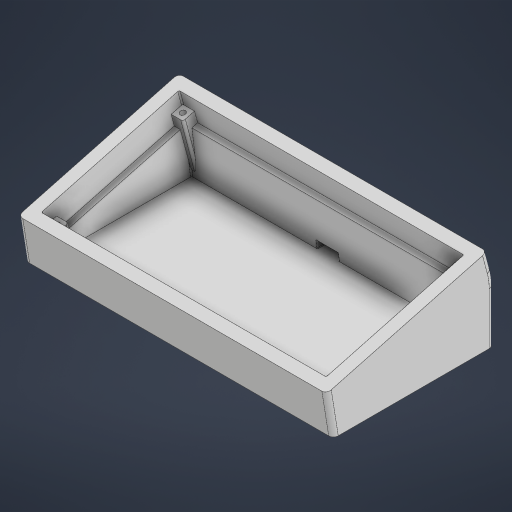
# Autodesk Inventor part: case
Saved by Autodesk Inventor 2024.2 (Build 282272000, 272)
## iProperties
Created: 2024-08-19
Part Number: case
Material: Generic
Document SubType Name: Modeling
Designer: Moe
Density: 1 g/cm^3
Appearance: Default
Author: Moe
Autodesk Inventor part; units mm, degrees
ref_plane "YZ Plane" through (0, 0, 0) normal (1, 0, 0) x (0, 1, 0)
ref_plane "XZ Plane" through (0, 0, 0) normal (0, 1, 0) x (-1, 0, 0)
sketch "Sketch1" plane through (0, 0, 0) normal (1, 0, 0) x (0, 1, 0)
  line L0 (0, 0) -> (7, 0)
  line L1 (7, 0) -> (25.1173, -67.6148)
  line L2 (25.1173, -67.6148) -> (0, -67.6148)
  line L3 (0, -67.6148) -> (0, 0)
  dimension "d0" = 7
  dimension "d1" = 70
  dimension "d2" = 105
  constraints: 8 end point, 1 horizontal, 1 parallel, 1 perpendicular
  measures "d0" distance of L0.start L0.end
  measures "d1" distance of L0.end L1.end
  measures "d2" angle of L0 L1
extrude "Extrusion1" add sketch "Sketch1" along normal blind 130
ref_plane "Work Plane1" through (0, 25, -67.6148) normal (0, -1, 0) x (1, 0, 0)
sketch "Sketch3" plane through (0, 7, 0) normal (0, 0.9659258, 0.258819) x (1, 0, 0)
  line L0 (5, 65) -> (125, 65)
  line L1 (125, 65) -> (125, 5)
  line L2 (125, 5) -> (5, 5)
  line L3 (5, 5) -> (5, 65)
  line L4 (0, 70) -> (130, 70) projected
  line L5 (0, 0) -> (130, 0) projected
  line L6 (0, 70) -> (0, 0) projected
  line L7 (130, 70) -> (130, 0) projected
  line L8 (5, 5) -> (10, 5)
  line L9 (10, 5) -> (10, 10)
  line L10 (10, 10) -> (5, 10)
  line L11 (5, 10) -> (5, 5)
  line L12 (5, 65) -> (10, 65)
  line L13 (10, 65) -> (10, 60)
  line L14 (10, 60) -> (5, 60)
  line L15 (5, 60) -> (5, 65)
  line L16 (125, 65) -> (120, 65)
  line L17 (120, 65) -> (120, 60)
  line L18 (120, 60) -> (125, 60)
  line L19 (125, 60) -> (125, 65)
  line L20 (125, 5) -> (120, 5)
  line L21 (120, 5) -> (120, 10)
  line L22 (120, 10) -> (125, 10)
  line L23 (125, 10) -> (125, 5)
  point P0 (0, -1.8117)
  point P1 (10, 5)
  dimension "d6" = 5
  dimension "d7" = 5
  dimension "d8" = 5
  dimension "d9" = 5
  dimension "d10" = 5
  dimension "d11" = 5
  dimension "d12" = 5
  dimension "d13" = 5
  dimension "d14" = 5
  dimension "d15" = 5
  dimension "d16" = 5
  dimension "d17" = 5
  constraints: 40 end point, 10 parallel, 5 horizontal, 5 perpendicular
  measures "d6" distance between parallel lines of L4 L0
  measures "d7" distance between parallel lines of L2 L5
  measures "d8" distance between parallel lines of L6 L3
  measures "d9" distance between parallel lines of L7 L1
  measures "d10" distance of L10.end L9.end
  measures "d11" distance of L9.end L8.end
  measures "d12" distance of L13.end L14.end
  measures "d13" distance of L12.end L13.end
  measures "d14" distance of L18.end L17.end
  measures "d15" distance of L17.end L16.end
  measures "d16" distance of L21.end L22.end
  measures "d17" distance of L20.end L21.end
sketch "Sketch4" plane through (0, 25, -67.6148) normal (0, -1, 0) x (1, 0, 0)
  line L0 (5, 57.9555) -> (5, 62.7852) projected
  line L1 (5, 62.7852) -> (5, 4.8296) projected
  line L2 (5, 62.7852) -> (10, 62.7852) projected
  line L3 (125, 62.7852) -> (5, 62.7852) projected
  line L4 (5, 4.8296) -> (125, 4.8296) projected
  line L5 (125, 4.8296) -> (125, 62.7852) projected
  point P0 (0, 67.6148)
extrude "Extrusion3" cut sketch "Sketch4" along normal blind 22
extrude "Extrusion4" add sketch "Sketch3" against normal blind 8 contours L10 L9 L2 L3 | L1 L2 L21 L22
sketch "Sketch5" plane through (10, 3, -6.2482) normal (1, 0, 0) x (0, 0, -1)
  line L0 (5.1764, 0) -> (0, 0) projected
  line L1 (0, 0) -> (-1.4185, 0)
  line L2 (-1.4185, 5.2941) -> (0, 0) projected
  line L3 (-1.4185, 0) -> (-1.4185, 5.2941)
  line L4 (-1.4185, 5.2941) -> (0, 0)
  point P0 (-6.2482, -3)
  constraints: 6 end point, 1 perpendicular
extrude "Extrusion5" add sketch "Sketch5" against normal blind 8
extrude "Extrusion6" add sketch "Sketch5" along normal blind 110
extrude "Extrusion7" add sketch "Sketch3" against normal blind 18 contours L0 L13 L14 L3 | L0 L1 L18 L17
extrude "Extrusion8" add sketch "Sketch3" along normal blind 5.1 contours L0 L13 L14 L3 | L0 L1 L18 L17 | L10 L9 L2 L3 | L1 L2 L21 L22
sketch "Sketch6" plane through (0, 7, 0) normal (0, 0.9659258, 0.258819) x (1, 0, 0)
  line L0 (7.5, 62.5) -> (122.5, 62.5)
  line L1 (122.5, 62.5) -> (122.5, 7.5)
  line L2 (122.5, 7.5) -> (7.5, 7.5)
  line L3 (7.5, 7.5) -> (7.5, 62.5)
  line L4 (10, 65) -> (120, 65) projected
  line L5 (5, 10) -> (5, 60) projected
  line L6 (120, 5) -> (10, 5) projected
  line L7 (125, 60) -> (125, 10) projected
  line L8 (5, 65) -> (5, 60) projected
  line L9 (120, 5) -> (125, 5) projected
  line L10 (5, 65) -> (125, 65)
  line L11 (125, 65) -> (125, 5)
  line L12 (125, 5) -> (5, 5)
  line L13 (5, 5) -> (5, 65)
  point P0 (0, -1.8117)
  point P1 (10, 5)
  point P2 (125, 10)
  dimension "d32" = 2.5
  dimension "d33" = 2.5
  dimension "d34" = 2.5
  dimension "d35" = 2.5
  constraints: 16 end point, 4 parallel, 2 horizontal, 2 perpendicular
  measures "d32" distance between parallel lines of L4 L0
  measures "d33" distance between parallel lines of L5 L3
  measures "d34" distance between parallel lines of L6 L2
  measures "d35" distance between parallel lines of L7 L1
extrude "Extrusion9" add sketch "Sketch6" against normal blind 8
sketch "Sketch7" plane through (5, 3, -62.7852) normal (1, 0, 0) x (0, 0, -1)
  line L0 (-2.7591, 11.8017) -> (-46.8038, 0) projected
  line L1 (-46.8038, 0) -> (0, 0) projected
  line L2 (0, 2.1883) -> (0, 0) projected
  line L3 (0, 2.1883) -> (-0.1709, 2.1425) projected
  line L4 (-0.1709, 2.1425) -> (-2.7591, 11.8017) projected
  point P0 (-62.7852, -3)
extrude "Extrusion10" add sketch "Sketch7" along normal blind 2.5
sketch "Sketch8" plane through (10, 5.1883, -62.7852) normal (1, 0, 0) x (0, 0, -1)
  line L0 (-0.3443, 10.2605) -> (-2.4148, 17.9879) projected
  line L1 (-2.4148, 17.9879) -> (0, -2.1883)
  line L2 (0, 10.3528) -> (-0.3443, 10.2605) projected
  line L3 (-0.3443, 10.2605) -> (-2.4148, 17.9879) projected
  line L4 (-2.4148, 17.9879) -> (0, 18.635) projected
  line L5 (0, 18.635) -> (-1.32, 23.5612) projected
  line L6 (-6.1496, 22.2671) -> (-1.32, 23.5612) projected
  line L7 (-6.1496, 22.2671) -> (-0.1709, -0.0458) projected
  line L8 (0, 0) -> (-0.1709, -0.0458) projected
  line L9 (0, 10.3528) -> (0, 0) projected
  line L10 (-0.1709, -0.0458) -> (0, -2.1883)
  line L11 (0, -2.1883) -> (0, 0)
  point P0 (-62.7852, -5.1883)
  point P1 (-0.3255, 0.5312)
  constraints: 6 end point, 1 vertical
extrude "Extrusion11" add sketch "Sketch8" against normal blind 2.5 contours L7 L10 L1 | L11 L10 L8
sketch "Sketch9" plane through (10, 3, -62.7852) normal (1, 0, 0) x (0, 0, -1)
  line L0 (0, 12.541) -> (-0.3443, 12.4488) projected
  line L1 (-0.3443, 12.4488) -> (-2.4148, 20.1762) projected
  line L2 (-2.4148, 20.1762) -> (0, 20.8232) projected
  line L3 (0, 20.8232) -> (-1.32, 25.7495) projected
  line L4 (-6.1496, 24.4554) -> (-1.32, 25.7495) projected
  line L5 (-6.1496, 24.4554) -> (-0.3255, 2.7194) projected
  line L6 (-0.3255, 2.7194) -> (0, 0) projected
  line L7 (0, 12.541) -> (0, 0) projected
  line L8 (-2.4148, 20.1762) -> (-4.8296, 19.5291)
  line L9 (-6.1496, 24.4554) -> (-0.3255, 2.7194) projected
  line L10 (-2.4148, 20.1762) -> (-0.3255, 2.7194)
  point P0 (-62.7852, -3)
  dimension "d42" = 2.5
  constraints: 4 end point, 1 collinear, 1 point on line
  measures "d42" distance of L1.end L8.end
extrude "Extrusion12" add sketch "Sketch9" along normal blind 110 contours L7 L6 L10 L1 L0
sketch "Sketch10" plane through (125, 3, -62.7852) normal (-1, 0, 0) x (0, 0, 1)
  line L0 (46.8038, 0) -> (2.7591, 11.8017) projected
  line L1 (2.7591, 11.8017) -> (0.1709, 2.1425) projected
  line L2 (0.1709, 2.1425) -> (0, 2.1883) projected
  line L3 (0, 2.1883) -> (0, 0) projected
  line L4 (0, 0) -> (46.8038, 0) projected
  point P0 (62.7852, -3)
extrude "Extrusion13" add sketch "Sketch10" along normal blind 2.5
fillet "Fillet1" radius 1 4 edges at (10, 16.5874, -59.5476) (10, 8.7572, -9.8819) (120, 16.5874, -59.5476) (120, 8.7572, -9.8819)
sketch "Sketch11" plane through (0, 7, 0) normal (0, 0.9659258, 0.258819) x (1, 0, 0)
  line L0 (5, 65) -> (10, 65) projected
  line L1 (125, 5) -> (125, 10) projected
  line L2 (5, 65) -> (125, 65)
  line L3 (125, 65) -> (125, 5)
  line L4 (125, 5) -> (5, 5)
  line L5 (5, 5) -> (5, 65)
  line L6 (0, 70) -> (0, 0) projected
  line L7 (0, 70) -> (130, 70) projected
  line L8 (0, 0) -> (130, 0) projected
  line L9 (130, 70) -> (130, 0) projected
  point P0 (0, -1.8117)
  constraints: 8 end point, 2 parallel, 1 horizontal, 1 perpendicular
extrude "Extrusion14" add sketch "Sketch11" along normal blind 11.1
sketch "Sketch12" plane through (130, 0, 0) normal (1, 0, 0) x (0, 0, -1)
  line L0 (-2.8729, 17.7218) -> (64.7419, 35.8391) projected
  line L1 (-2.8729, 17.7218) -> (0, 0)
  line L2 (0, 7) -> (-2.8729, 17.7218) projected
  line L3 (0, 0) -> (0, 7)
  line L4 (0, 7) -> (-2.8729, 17.7218)
  constraints: 6 end point, 1 collinear, 1 vertical
extrude "Extrusion15" add sketch "Sketch12" against normal blind 130
fillet "Fillet2" radius 25 1 edges at (65, 25.1173, -67.6148)
fillet "Fillet3" radius 2 8 edges at (130, 8.8609, 1.4364) (130, 10.913, -67.6148) (130, 32.0678, -65.7524) (130, 25.0892, -67.4009) (0, 8.8609, 1.4364) (0, 25.0892, -67.4009) (0, 32.0678, -65.7524) (0, 10.913, -67.6148)
fillet "Fillet4" radius 0.5 4 edges at (5, 31.6472, -60.6887) (125, 31.6472, -60.6887) (5, 16.1181, -2.7332) (125, 16.1181, -2.7332)
fillet "Fillet5" radius 0.5 6 edges at (7.5, 6.2941, -10.5419) (10, 5.9706, -8.0404) (7.5, 4.3597, -62.6224) (122.5, 4.0941, -62.7852) (122.5, 6.2941, -10.5419) (120, 5.9706, -8.0404)
sketch "Sketch13" plane through (128, 21.826, -67.6148) normal (0, 0, -1) x (-1, 0, 0)
  line L0 (120, -18.826) -> (120, -16.1066) projected
  line L1 (120, -18.826) -> (8, -18.826) projected
  line L2 (8, -16.1066) -> (8, -18.826) projected
  line L3 (8, -16.1066) -> (7, -16.1066) projected
  ellipse E0 centre (7, -9.1239) end of major axis (7, -16.1066) minor radius 1 (7, -16.1066) -> (8, -9.1239) ccw projected
  line L4 (8, 1.3502) -> (8, -9.1239) projected
  line L5 (118, 1.3502) -> (8, 1.3502) projected
  line L6 (118, -9.1239) -> (118, 1.3502) projected
  ellipse E1 centre (119, -9.1239) end of major axis (119, -2.1412) minor radius 1 (118, -9.1239) -> (119, -16.1066) ccw projected
  line L7 (120, -16.1066) -> (119, -16.1066) projected
  line L8 (58.25, -15.326) -> (67.75, -15.326)
  line L9 (67.75, -15.326) -> (67.75, -18.826)
  line L10 (67.75, -18.826) -> (58.25, -18.826)
  line L11 (58.25, -18.826) -> (58.25, -15.326)
  line L12 (128, -21.826) -> (128, 0) projected
  point P0 (63, -15.326)
  dimension "d56" = 9.5
  dimension "d57" = 3.5
  dimension "d58" = 0
  dimension "d59" = 65
  constraints: 8 end point, 2 parallel, 1 horizontal, 1 midpoint, 1 perpendicular, 2 other
  measures "d56" distance of L9.end L10.end
  measures "d57" distance of L8.end L9.end
  measures "d58" distance between parallel lines of L1 L10
  measures "d59" distance from line of L12 point (63, -15.326)
extrude "Extrusion16" cut sketch "Sketch13" against normal blind 8 contours L1 L11 L8 L9
fillet "Fillet6" radius 0.25 4 edges at (60.25, 6.5, -64.9905) (69.75, 3, -65.2) (60.25, 3, -65.2) (69.75, 6.5, -64.9905)
sketch "Sketch14" plane through (0, 11.9262, 1.32) normal (0, 0.9659258, 0.258819) x (1, 0, 0)
  line L0 (10, 61) -> (10, 65) projected
  arc A0 (5.5, 65) -> (5, 64.5) centre (5.5, 64.5) ccw projected
  line L1 (5, 64.5) -> (5, 60) projected
  line L2 (5, 60) -> (9, 60) projected
  arc A1 (9, 60) -> (10, 61) centre (9, 61) ccw projected
  line L3 (10, 61) -> (10, 65) projected
  line L4 (10, 65) -> (5.5, 65) projected
  arc A2 (125, 64.5) -> (124.5, 65) centre (124.5, 64.5) ccw projected
  line L5 (124.5, 65) -> (120, 65) projected
  line L6 (120, 65) -> (120, 61) projected
  arc A3 (120, 61) -> (121, 60) centre (121, 61) ccw projected
  line L7 (121, 60) -> (125, 60) projected
  line L8 (125, 60) -> (125, 64.5) projected
  arc A4 (124.5, 5) -> (125, 5.5) centre (124.5, 5.5) ccw projected
  line L9 (125, 5.5) -> (125, 10) projected
  line L10 (125, 10) -> (121, 10) projected
  arc A5 (121, 10) -> (120, 9) centre (121, 9) ccw projected
  line L11 (120, 9) -> (120, 5) projected
  line L12 (120, 5) -> (124.5, 5) projected
  arc A6 (5, 5.5) -> (5.5, 5) centre (5.5, 5.5) ccw projected
  line L13 (5.5, 5) -> (10, 5) projected
  line L14 (10, 5) -> (10, 9) projected
  arc A7 (10, 9) -> (9, 10) centre (9, 9) ccw projected
  line L15 (9, 10) -> (5, 10) projected
  line L16 (5, 10) -> (5, 5.5) projected
  circle A8 centre (7.5, 62.5) radius 1.1
  circle A9 centre (122.5, 62.5) radius 1.1
  circle A10 centre (122.5, 7.5) radius 1.1
  circle A11 centre (7.5, 7.5) radius 1.1
  point P0 (0, -1.8117)
  point P1 (122.25, 5)
  dimension "d63" = 2.2
  dimension "d64" = 2.2
  dimension "d65" = 2.2
  dimension "d66" = 2.2
  dimension "d67" = 2.5
  dimension "d68" = 2.5
  dimension "d69" = 2.5
  dimension "d70" = 2.5
  dimension "d71" = 2.5
  dimension "d72" = 2.5
  dimension "d73" = 2.5
  dimension "d74" = 2.5
  constraints: 4 centre point, 1 midpoint
  measures "d63" diameter of A8
  measures "d64" diameter of A9
  measures "d65" diameter of A10
  measures "d66" diameter of A11
  measures "d67" distance from line of L0 A8.centre
  measures "d68" distance from line of L2 A8.centre
  measures "d69" distance from line of L7 A9.centre
  measures "d70" distance from line of L6 A9.centre
  measures "d71" distance from line of L11 A10.centre
  measures "d72" vertical distance of A10.centre point (122.25, 5)
  measures "d73" distance from line of L14 A11.centre
  measures "d74" distance from line of L13 A11.centre
extrude "Extrusion17" cut sketch "Sketch14" against normal blind 12 contours A8 | A9 | A10 | A11
body "Solid1"
